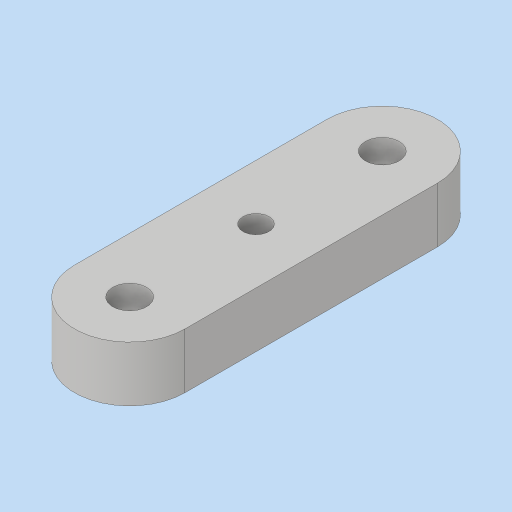
# Autodesk Inventor part: futek-holder
Saved by Autodesk Inventor 2024 (Build 280153000, 153)
## iProperties
Created: 2023-04-24
Part Number: futek-holder
Material: Generic
Document SubType Name: Modeling
Designer: Karbosch
Mass: 3.89321 g
Surface Area: 21.7139 cm^2
Volume: 3.89321 cm^3
Density: 1 g/cm^3
Appearance: Default
Author: Karbosch
Autodesk Inventor part; units mm, degrees
ref_plane "YZ Plane" through (0, 0, 0) normal (1, 0, 0) x (0, 1, 0)
ref_plane "XZ Plane" through (0, 0, 0) normal (0, 1, 0) x (-1, 0, 0)
ref_plane "XY Plane" through (0, 0, 0) normal (0, 0, 1) x (1, 0, 0)
sketch "Sketch1" plane through (0, 0, 0) normal (0, 1, 0) x (-1, 0, 0)
  circle A0 centre (0, 0) radius 1.65
  line L0 (0, 0) -> (0, -16) construction
  line L1 (-7, 0) -> (-7, -16)
  line L2 (7, -16) -> (7, 0)
  arc A1 (7, 0) -> (-7, 0) centre (0, 0) ccw
  arc A2 (-7, -16) -> (7, -16) centre (0, -16) ccw
  circle A3 centre (0, -16) radius 2.15
  point P0 (0, -8)
  dimension "d0" = 3.3
  dimension "d1" = 16
  dimension "d2" = 14
  dimension "d3" = 4.3
  constraints: 8 end point, 4 centre point, 4 point on circle, 4 tangent, 2 coincident, 1 midpoint, 1 parallel, 1 vertical
  measures "d0" diameter of A0
  measures "d1" distance of L0.start L0.end
  measures "d2" diameter of A2
  measures "d3" diameter of A3
extrude "Extrusion1" add sketch "Sketch1" along normal blind 7
sketch "Sketch2" plane through (0, 0, 0) normal (0, -1, 0) x (1, 0, 0)
  circle A0 centre (0, 0) radius 1.65 projected
  circle A1 centre (0, 0) radius 2.9
  dimension "d6" = 5.8
  constraints: 1 centre point, 1 coincident
  measures "d6" diameter of A1
extrude "Extrusion2" cut sketch "Sketch2" against normal blind 3.2
mirror "Mirror1" about plane through (0, 0, 0) normal (0, 0, 1) of "Extrusion1", "Extrusion2"
ref_plane "Work Plane1" through (0, 0, 0) normal (0, 0, 1) x (1, 0, 0)
body "Solid1"
